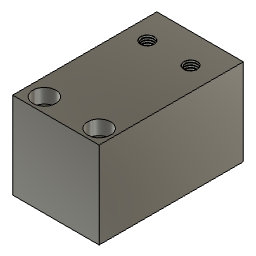
02 (Autodesk Fusion 360 design; units mm, degrees)
Autodesk Fusion 360 part; units mm, degrees
sketch "Sketch2" plane through (0, 0, 0) normal (0, 0, 1) x (1, 0, 0)
  line L0 (0, 0) -> (30, 0)
  line L1 (30, 0) -> (30, 50)
  line L2 (30, 50) -> (0, 50)
  line L3 (0, 50) -> (0, 0)
  dimension "d5" = 30
  dimension "d6" = 50
  constraint horizontal L0
  constraint vertical L1
  constraint horizontal L2
  constraint vertical L3
  constraint coincident L0.start L3.end
  measures "d5" distance of L0.start L0.end
  measures "d6" distance of L0.start L2.end
extrude "Extrude2" add sketch "Sketch2" along normal blind 30
hole "Hole1" at (20, 38, 30) direction (0, 0, -1) diameter 2.4 end through all
delete_face "DeleteFace1" 1 faces at (20.1195, 36.806, 20)
sketch "Sketch3" plane through (0, 0, 30) normal (0, 0, 1) x (-1, 0, 0)
  line L0 (0, -50) -> (0, 0)
  line L1 (-6, -5) -> (-25, -5)
  line L2 (0, 0) -> (-30, 0)
  line L3 (-30, 0) -> (-30, -50)
  dimension "d12" = 5
  dimension "d13" = 5
  constraint perpendicular L0 L1
  measures "d12" distance of L1 L2
  measures "d13" distance of L1.end L3
hole "Hole2" at (25, 5, 30) at (6, 5, 30) direction (0, 0, -1) diameter 5 end through all counterbore diameter 8 counterbore depth 5
sketch "Sketch4" plane through (0, 0, 30) normal (0, 0, 1) x (-1, 0, 0)
  line L0 (-7, -40) -> (-22, -40)
  line L1 (-30, -50) -> (0, -50)
  dimension "d19" = 10
  dimension "d20" = 15
  measures "d19" distance of L0 L1
  measures "d20" distance of L0.start L0.end
hole "Hole4" at (7, 40, 30) at (22, 40, 30) direction (0, 0, -1) diameter 4.234 depth 10 tip angle 118
thread "Thread2" "ISO Metric profile 5.0 M5x0.8 6H" major diameter 5.12 minor diameter 4.234 pitch 0.8 angle 60 modelled right hand crest width 0.2219 on face at (7.1055, 37.8856, 26.6667) crest through (9.117, 40, 29.8) on face at (19.8837, 40.0528, 26.6667) crest through (24.117, 40, 29.8)
hole "Hole3" [rolled back] hole depth 10 hole diameter 4.234 tip angle 118
thread "Thread1" "ISO Metric profile 5.0 M5x0.8 6H"
sketch "Sketch1" plane through (0, 0, 0) normal (0, 0, 1) x (1, 0, 0)
  line L0 (-30, 50) -> (0, 50)
  line L1 (0, 50) -> (0, 0)
  line L2 (0, 0) -> (-30, 0)
  line L3 (-30, 0) -> (-30, 50)
  dimension "d1" = 30
  dimension "d2" = 50
  constraint horizontal L0
  constraint vertical L1
  constraint horizontal L2
  constraint vertical L3
  measures "d1" distance of L0.start L0.end
  measures "d2" distance of L0.start L2.end
extrude "Extrude1" [rolled back] along distance 10 taper angle 0
